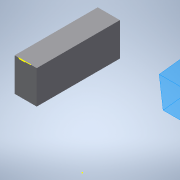
# Autodesk Inventor part: structure_core_cradle
Saved by Autodesk Inventor 2020.2 (Build 242310000, 310)
## iProperties
Created: 2020-06-29
Part Number: structure_core_cradle
Material: 一般
Document SubType Name: Modeling
Designer: gisen
Density: 1 g/cm^3
Appearance: 既定
Author: gisen
Autodesk Inventor part; units mm, degrees
ref_plane "YZ Plane" through (0, 0, 0) normal (1, 0, 0) x (0, 1, 0)
ref_plane "XZ Plane" through (0, 0, 0) normal (0, 1, 0) x (-1, 0, 0)
ref_plane "XY Plane" through (0, 0, 0) normal (0, 0, 1) x (1, 0, 0)
sketch "スケッチ1" plane through (0, 0, 0) normal (0, 0, 1) x (1, 0, 0)
  line L0 (-122.1591, 122.1591) -> (-82.1591, 122.1591)
  line L1 (-82.1591, 122.1591) -> (-82.1591, 67.1591)
  line L2 (-82.1591, 67.1591) -> (-122.1591, 67.1591)
  line L3 (-122.1591, 67.1591) -> (-122.1591, 122.1591)
  point P0 (0, 0)
  dimension "d0" = 40
  dimension "d1" = 55
  constraints: 8 end point, 2 parallel, 1 horizontal, 1 perpendicular
  measures "d0" distance of L0.start L0.end
  measures "d1" distance of L2.end L0.start
extrude "押し出し1" add sketch "スケッチ1" along normal blind 150
sketch "スケッチ4" plane through (0, 0, 150) normal (0, 0, 1) x (1, 0, 0)
  line L0 (-82.1591, 122.1591) -> (-122.1591, 122.1591) projected
  line L1 (-117.1591, 101.5897) -> (-92.1591, 101.5897)
  line L2 (-92.1591, 101.5897) -> (-92.1591, 122.1591)
  line L3 (-92.1591, 122.1591) -> (-117.1591, 122.1591)
  line L4 (-117.1591, 122.1591) -> (-117.1591, 101.5897)
  line L5 (-82.1591, 67.1591) -> (-82.1591, 122.1591) projected
  point P0 (0, 0)
  dimension "d4" = 10
  dimension "d5" = 25
  constraints: 8 end point, 2 parallel, 1 horizontal, 1 perpendicular, 1 point on line
  measures "d4" distance between parallel lines of L5 L2
  measures "d5" distance of L1.start L1.end
extrude "押し出し2" cut sketch "スケッチ4" against normal blind 21.4
sketch "スケッチ5" plane through (0, 0, 150) normal (0, 0, 1) x (1, 0, 0)
  line L0 (-116.288, 107.2289) -> (-115.2421, 122.1591) projected
  line L1 (-93.2061, 122.1591) -> (-92.1591, 107.2289) projected
  line L2 (-95.5428, 103.9291) -> (-112.9179, 103.9291) projected
  line L3 (-115.2421, 122.1591) -> (-93.2061, 122.1591) projected
  line L4 (-112.2468, 103.9291) -> (-108.7036, 103.9291) projected
  line L5 (-95.5428, 103.9291) -> (-112.9179, 103.9291) projected
  line L6 (-92.1591, 104.7291) -> (-92.1591, 104.7291)
  line L7 (-116.2893, 104.7291) -> (-116.288, 103.9291)
  line L8 (-116.288, 103.9291) -> (-114.2025, 103.9291)
  line L9 (-92.1591, 104.7291) -> (-92.1591, 103.9291)
  line L10 (-95.5428, 103.9291) -> (-92.1591, 103.9291)
  line L11 (-114.2025, 103.9291) -> (-112.9179, 103.9291)
  line L12 (-116.2893, 104.7291) -> (-116.288, 103.9291)
  line L13 (-116.288, 103.9291) -> (-112.9179, 103.9291)
  line L14 (-92.1591, 104.7291) -> (-92.1591, 103.9291)
  line L15 (-95.5428, 103.9291) -> (-92.1591, 103.9291)
  line L16 (-92.1591, 103.9291) -> (-92.1591, 107.2289)
  line L17 (-92.1591, 103.9291) -> (-95.5428, 103.9291)
  line L18 (-95.5428, 103.9291) -> (-116.288, 103.9291)
  line L19 (-116.288, 103.9291) -> (-116.288, 104.7291)
  line L20 (-116.288, 107.2289) -> (-116.288, 104.7291)
  point P0 (0, 0)
  constraints: 30 end point, 4 collinear, 2 perpendicular, 2 vertical, 1 horizontal
extrude "押し出し3" cut sketch "スケッチ5" against normal blind 130
sketch "スケッチ6" plane through (0, 0, 150) normal (0, 0, 1) x (1, 0, 0)
  line L0 (-122.1591, 67.1591) -> (-82.1591, 67.1591) projected
  line L1 (-122.1591, 67.1591) -> (-97.1591, 67.1591)
  line L2 (-97.1591, 67.1591) -> (-97.1591, 97.1591)
  line L3 (-97.1591, 97.1591) -> (-122.1591, 97.1591)
  line L4 (-122.1591, 97.1591) -> (-122.1591, 67.1591)
  line L5 (-82.1591, 67.1591) -> (-82.1591, 122.1591) projected
  point P0 (0, 0)
  dimension "d10" = 30
  dimension "d11" = 15
  constraints: 8 end point, 2 parallel, 1 horizontal, 1 perpendicular
  measures "d10" distance of L1.end L2.end
  measures "d11" distance between parallel lines of L5 L2
extrude "押し出し4" cut sketch "スケッチ6" against normal blind 170
sketch "スケッチ7" plane through (-82.1591, 67.1591, 0) normal (1, 0, 0) x (0, 0, -1)
  circle A0 centre (-140.2625, 35) radius 1.65
  circle A1 centre (-107.2625, 13) radius 1.65
  circle A2 centre (-45.2625, 13) radius 1.65
  circle A3 centre (-12.2625, 35) radius 1.65
  point P0 (0, -67.1591)
  dimension "d14" = 3.3
  dimension "d15" = 3.3
  dimension "d16" = 3.3
  dimension "d17" = 3.3
  constraints: 4 centre point
  measures "d14" diameter of A0
  measures "d15" diameter of A1
  measures "d16" diameter of A2
  measures "d17" diameter of A3
extrude "押し出し5" cut sketch "スケッチ7" against normal blind 5
fillet "フィレット1" radius 2 26 edges at (-122.1591, 109.6591, 0) (-122.1591, 97.1591, 75) (-122.1591, 122.1591, 75) (-102.1591, 122.1591, 0) (-122.1591, 109.6591, 150) (-119.6591, 122.1591, 150) (-117.1591, 111.8744, 150) (-92.1591, 102.7594, 150) (-92.1591, 114.694, 150) (-87.1591, 122.1591, 150) (-92.1591, 122.1591, 139.3) (-104.6591, 101.5897, 150) (-109.6591, 97.1591, 150) (-97.1591, 82.1591, 150) (-97.1591, 67.1591, 75) (-89.6591, 67.1591, 150) (-97.1591, 82.1591, 0) (-89.6591, 67.1591, 0) (-97.1591, 97.1591, 75) (-109.6591, 97.1591, 0) (-104.2241, 122.1591, 20) (-117.1591, 122.1591, 139.3) (-116.2006, 122.1591, 128.6) (-92.6826, 122.1591, 128.6) (-115.2421, 122.1591, 74.3) (-93.2061, 122.1591, 74.3)
